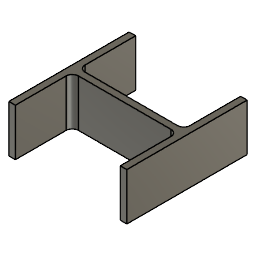
H-200×204×12×12 (Autodesk Fusion 360 design; units mm, degrees)
Autodesk Fusion 360 part; units mm, degrees
sketch "スケッチ1" plane through (0, 0, 0) normal (0, 0, 1) x (1, 0, 0)
  line L0 (0, 127.5) -> (0, -127.5)
  line L1 (250, -127.5) -> (250, 127.5)
  line L2 (236, -20) -> (236, -127.5)
  line L3 (14, -127.5) -> (14, -20)
  line L4 (0, -127.5) -> (14, -127.5)
  line L5 (236, -127.5) -> (250, -127.5)
  line L6 (14, 20) -> (14, 127.5)
  line L7 (236, 127.5) -> (236, 20)
  line L8 (223, 7) -> (27, 7)
  line L9 (27, -7) -> (223, -7)
  line L10 (14, 127.5) -> (0, 127.5)
  line L11 (250, 127.5) -> (236, 127.5)
  arc A0 (27, -7) -> (14, -20) centre (27, -20) ccw
  arc A1 (14, 20) -> (27, 7) centre (27, 20) ccw
  arc A2 (223, 7) -> (236, 20) centre (223, 20) ccw
  arc A3 (236, -20) -> (223, -7) centre (223, -20) ccw
extrude "押し出し1" add sketch "スケッチ1" along normal blind 100
